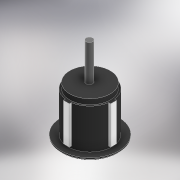
# Autodesk Inventor part: JSN-SR04 US Sensor
Saved by Autodesk Inventor 2021 (Build 250183000, 183)
## iProperties
Created: 2021-01-11
Part Number: JSN-SR04 US Sensor
Material: ABS-Kunststoff
Document SubType Name: Modeling
Designer: rth
Density: 1.06 g/cm^3
Appearance: Gummi - Schwarz
Author: rth
Autodesk Inventor part; units mm, degrees
ref_plane "YZ Plane" through (0, 0, 0) normal (1, 0, 0) x (0, 1, 0)
ref_plane "XZ Plane" through (0, 0, 0) normal (0, 1, 0) x (-1, 0, 0)
ref_plane "XY Plane" through (0, 0, 0) normal (0, 0, 1) x (1, 0, 0)
sketch "Skizze1" plane through (0, 0, 0) normal (0, 1, 0) x (-1, 0, 0)
  circle A0 centre (0, 0) radius 9
  dimension "d0" = 18
  constraints: 1 centre point, 1 coincident
  measures "d0" diameter of A0
extrude "Extrusion1" add sketch "Skizze1" along normal blind 16.34
sketch "Skizze2" plane through (0, 16.34, 0) normal (0, 1, 0) x (1, 0, 0)
  circle A0 centre (0, 0) radius 8.3
  dimension "d3" = 16.6
  constraints: 1 centre point, 1 coincident
  measures "d3" diameter of A0
extrude "Extrusion2" add sketch "Skizze2" along normal blind 2.16
sketch "Skizze3" plane through (0, 0, 0) normal (0, -1, 0) x (1, 0, 0)
  circle A0 centre (0, 0) radius 11.875
  dimension "d6" = 23.75
  constraints: 1 centre point, 1 coincident
  measures "d6" diameter of A0
extrude "Extrusion3" add sketch "Skizze3" along normal blind 2
sketch "Skizze4" plane through (0, -2, 0) normal (0, -1, 0) x (1, 0, 0)
  circle A0 centre (0, 0) radius 7.075
  circle A1 centre (0, 0) radius 8.5
  dimension "d9" = 14.15
  dimension "d10" = 17
  constraints: 2 centre point, 2 coincident
  measures "d9" diameter of A0
  measures "d10" diameter of A1
extrude "Extrusion4" cut sketch "Skizze4" against normal blind 1
fillet "Rundung1" radius 0.25 2 edges at (-7.075, -2, 0) (-8.5, -2, 0)
sketch "Skizze5" plane through (0, 0, 0) normal (1, 0, 0) x (0, 1, 0)
  line L0 (-2, 11.875) -> (-2, -11.875) projected
  line L1 (0, 11.875) -> (-2, 11.875) projected
  arc A0 (-0.5, 11.875) -> (-2, 8.9956) centre (1.5136, 8.9956) ccw
  line L2 (0, 0) -> (-4.6348, 0)
  dimension "d14" = 0.5
  constraints: 2 end point, 2 point on circle, 2 point on line, 1 centre point, 1 horizontal, 1 tangent
  measures "d14" distance of L1.start A0.start
revolve "Umdrehung1" cut sketch "Skizze5" angle 360 about axis through (0, 0, 0) along (0, -1, 0)
sketch "Skizze6" plane through (0, 16.34, 0) normal (0, 1, 0) x (1, 0, 0)
  line L0 (-8.2456, -1.2678) -> (-9.7456, -1.2678)
  line L1 (-9.7456, -1.2678) -> (-9.7456, 1.2678)
  line L2 (-9.7456, 1.2678) -> (-8.2456, 1.2678)
  line L3 (-8.2456, 1.2678) -> (-8.2456, -1.2678)
  circle A0 centre (0, 0) radius 8.9956 projected
  line L4 (-8.2456, -1.2678) -> (-9.7456, 1.2678) construction
  line L5 (-9.7456, -1.2678) -> (-8.2456, 1.2678) construction
  point P0 (-8.9956, 0)
  dimension "d16" = 0.75
  constraints: 12 end point, 2 midpoint, 2 parallel, 1 horizontal, 1 horizontal alignment, 1 perpendicular, 1 other
  measures "d16" distance from line of point (-8.996, 0) L1
extrude "Extrusion5" add sketch "Skizze6" against normal blind 15.5 contours L0 A0 L2 L3 | L0 L1 L2 A0 picked at (-8.4923, -0.1413)
fillet "Rundung2" radius 0.1 2 edges at (-9.7456, 8.59, -1.2678) (-9.7456, 8.59, 1.2678)
pattern_circular "Runde Anordnung1" count 4 over 360 about axis through (0, 0, 0) along (0, 1, 0) of "Extrusion5", "Rundung2"
sketch "Skizze7" plane through (0, 18.5, 0) normal (0, 1, 0) x (1, 0, 0)
  circle A0 centre (-0.2666, 0) radius 1.375
  point P0 (0, 0)
  dimension "d23" = 2.75
  constraints: 1 centre point
  measures "d23" diameter of A0
extrude "Extrusion6" add sketch "Skizze7" along normal blind 15
